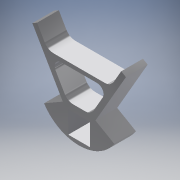
# Autodesk Inventor part: vertex-01
Saved by Autodesk Inventor 2016 (Build 200138000, 138)
## iProperties
Created: 2015-08-21
Part Number: vertex-01
Material: Aluminum 6061
Document SubType Name: Modeling
Designer: ubik
Density: 2.7 g/cm^3
Appearance: Aluminum - Polished
Author: ubik
Autodesk Inventor part; units mm, degrees
ref_plane "YZ Plane" through (0, 0, 0) normal (1, 0, 0) x (0, 1, 0)
ref_plane "XZ Plane" through (0, 0, 0) normal (0, 1, 0) x (-1, 0, 0)
ref_plane "XY Plane" through (0, 0, 0) normal (0, 0, 1) x (1, 0, 0)
sketch "Sketch1" plane through (0, 0, 0) normal (0, 0, 1) x (1, 0, 0)
  line L0 (-60.4663, 57.5499) -> (-26.2078, -1.7874) construction
  line L1 (60.5489, 57.6931) -> (26.7783, -0.7993) construction
  line L2 (-46.1983, -8.6) -> (53.905, -8.6) construction
  line L3 (-43, 67.2974) -> (-15, 18.8)
  line L4 (43, 67.2974) -> (15, 18.8)
  line L5 (15, 18.8) -> (32.2735, 8.8271)
  line L6 (-15, 18.8) -> (-32.2735, 8.8271)
  line L7 (-43, 67.2974) -> (-38.6699, 69.7974)
  line L8 (38.6699, 69.7974) -> (43, 67.2974)
  line L9 (-10, 15) -> (10, 15)
  line L10 (10, 15) -> (10, -5)
  line L11 (10, -5) -> (-10, -5)
  line L12 (-10, -5) -> (-10, 15)
  line L13 (-38.6699, 69.7974) -> (-31.7143, 57.75)
  line L14 (38.6699, 69.7974) -> (31.7143, 57.75)
  line L15 (10.7276, 21.4) -> (10.6699, 21.3)
  line L16 (-5.5315, 21.4) -> (5.5315, 21.4)
  arc A0 (-32.2735, 8.8271) -> (32.2735, 8.8271) centre (0, 29.8192) ccw
  arc A1 (-33.342, 10.5692) -> (-32.2735, 8.8271) centre (0, 29.8192) ccw
  line L17 (-16.5011, 49.4) -> (16.5011, 49.4)
  line L18 (-23.4871, 53) -> (23.4871, 53)
  line L19 (-21.6973, 40.4) -> (-13.3257, 25.9)
  line L20 (21.6973, 40.4) -> (13.3257, 25.9)
  arc A2 (-31.7143, 57.75) -> (-23.4871, 53) centre (-23.4871, 62.5) ccw
  arc A3 (23.4871, 53) -> (31.7143, 57.75) centre (23.4871, 62.5) ccw
  arc A4 (-13.3257, 25.9) -> (-5.5315, 21.4) centre (-5.5315, 30.4) ccw
  arc A5 (5.5315, 21.4) -> (13.3257, 25.9) centre (5.5315, 30.4) ccw
  arc A6 (-16.5011, 49.4) -> (-21.6973, 40.4) centre (-16.5011, 43.4) ccw
  arc A7 (21.6973, 40.4) -> (16.5011, 49.4) centre (16.5011, 43.4) ccw
  point P0 (0, 0)
  point P1 (-10.7276, 21.4)
  point P2 (-26.8934, 49.4)
  point P3 (26.8934, 49.4)
  dimension "d12" = 30
  dimension "d13" = 15
  dimension "d15" = 20
  dimension "d16" = 20
  dimension "d20" = 56
  dimension "d21" = 56
  dimension "d22" = 20
  dimension "d23" = 20
  dimension "d24" = 10
  dimension "d31" = 15
  dimension "d33" = 77
  dimension "d34" = 30
  dimension "d37" = 28
  dimension "d38" = 5
  dimension "d39" = 5
  dimension "d40" = 3.6
  dimension "d41" = 9.5
  dimension "d42" = 9
  dimension "d43" = 6
  constraints: 42 end point, 16 point on circle, 14 tangent, 12 point on line, 8 centre point, 6 parallel, 5 perpendicular, 4 horizontal, 3 equal radius, 2 other
  measures "d12" distance of L3.end L4.end
  measures "d13" horizontal distance of point (0, 0) L3.end
  measures "d15" distance between parallel lines of L1 L4
  measures "d16" distance between parallel lines of L3 L0
  measures "d20" distance between parallel lines of L5 L8
  measures "d21" distance between parallel lines of L6 L7
  measures "d22" distance of L9.start L9.end
  measures "d23" distance of L11.end L9.start
  measures "d24" distance from line of point (0, 0) L12
  measures "d31" distance from line of point (0, 0) L9
  measures "d33" diameter of A0
  measures "d34" distance between parallel lines of L2 L16
  measures "d37" distance between parallel lines of L16 L17
  measures "d38" distance between parallel lines of L3 L13
  measures "d39" distance between parallel lines of L4 L14
  measures "d40" distance between parallel lines of L17 L18
  measures "d41" radius of A2
  measures "d42" radius of A4
  measures "d43" radius of A6
extrude "Extrusion2" add sketch "Sketch1" along normal blind 20 contours L7 L13 A2 L18 A3 L14 L8 L4 L5 A0 L6 L3 | A4 L19 A6 L17 A7 L20 A5 L16
extrude "Extrusion3" cut sketch "Sketch1" along normal through all contours A4 L19 A6 L17 A7 L20 A5 L16
equation "\"d13\" = 0.5 * d12"
equation "\"d23\" = d22"
equation "\"d24\" = 0.5 * d22"
equation "\"d39\" = d38"
body "Solid2"
